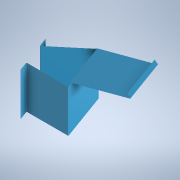
# Autodesk Inventor part: Silla2
Saved by Autodesk Inventor 2022 (Build 260153000, 153)
## iProperties
Created: 2023-10-21
Part Number: Silla2
Material: Generic
Document SubType Name: Sheet Metal
Designer: Administrador
Density: 1 g/cm^3
Sheet Metal Rule: Default
Appearance: Sky Blue Dark
Flat Pattern Width: 113.2 cm
Flat Pattern Length: 180 cm
Flat Pattern Area: 20376 cm^2
Sheet Metal Width: 1132.000 mm
Sheet Metal Length: 1800.000 mm
Sheet Metal Area: 2037600.000 mm^2
Author: Administrador
Autodesk Inventor part; units mm, degrees
ref_plane "YZ Plane" through (0, 0, 0) normal (1, 0, 0) x (0, 1, 0)
ref_plane "XZ Plane" through (0, 0, 0) normal (0, 1, 0) x (-1, 0, 0)
ref_plane "XY Plane" through (0, 0, 0) normal (0, 0, 1) x (1, 0, 0)
sketch "Sketch1" plane through (0, 0, 0) normal (0, 0, 1) x (1, 0, 0)
  point P0 (0, 0)
sketch "Sketch2" plane through (0, 0, 0) normal (0, 0, 1) x (1, 0, 0)
  line L0 (0, 0) -> (1800, 0)
  line L1 (1800, 0) -> (1800, 500)
  line L2 (1800, 500) -> (0, 500)
  line L3 (0, 500) -> (0, 0)
  line L4 (900, 500) -> (900, 0)
  line L5 (900, 500) -> (1170, 500)
  line L6 (1170, 500) -> (630, 500)
  line L7 (630, 500) -> (630, 1132)
  line L8 (630, 1132) -> (1170, 1132)
  line L9 (1170, 1132) -> (1170, 500)
  line L10 (630, 500) -> (630, 520)
  line L11 (630, 520) -> (610, 520)
  arc A0 (610, 500) -> (630, 520) centre (610, 520) ccw
  arc A1 (1170, 520) -> (1190, 500) centre (1190, 520) ccw
  line L12 (610, 500) -> (630, 500)
  line L13 (630, 520) -> (630, 500)
  line L14 (1170, 520) -> (1170, 500)
  line L15 (1190, 500) -> (1170, 500)
  dimension "d0" = 1800
  dimension "d1" = 500
  dimension "d32" = 270
  dimension "d33" = 540
  dimension "d34" = 632
  dimension "d49" = 20
  dimension "d50" = 20
  measures "d0" distance of L0.start L0.end
  measures "d1" distance of L0.end L1.end
  measures "d32" distance of L4.start L5.end
  measures "d33" distance of L7.end L8.end
  measures "d34" distance of L6.end L7.end
  measures "d49" distance of L6.end L10.end
  measures "d50" distance of L10.end L11.end
extrude "Plate1" add sketch "Sketch2" along normal blind 3.048
sketch "Sketch3" plane through (0, 0, 3.048) normal (0, 0, 1) x (1, 0, 0)
  line L0 (1800, 500) -> (0, 500) projected
  line L1 (900, 500) -> (900, 0)
  line L2 (0, 0) -> (1800, 0) projected
  line L3 (900, 0) -> (600, 0)
  line L4 (600, 0) -> (600, 500)
  line L5 (600, 0) -> (110, 0)
  line L6 (0, 500) -> (0, 0) projected
  line L7 (110, 0) -> (0, 0)
  line L8 (110, 0) -> (110, 500)
  line L9 (1200, 0) -> (1200, 500)
  line L10 (1690, 0) -> (1690, 500)
  dimension "d3" = 300
  dimension "d4" = 490
  constraints: 16 end point, 4 symmetric about line, 3 perpendicular, 2 midpoint, 2 point on line, 1 collinear
  measures "d3" distance of L1.end L3.end
  measures "d4" distance of L3.end L5.end
fold "Fold1" angle 110 bend radius 3.048 thickness 3.048 k factor 0.44 line from (110, 0, 3.048) to (110, 500, 3.048) line at bend centre moving side (-1, 0, 0) folds toward (0, 0, 1)
fold "Fold2" angle 110 bend radius 3.048 thickness 3.048 k factor 0.44 line from (600, 0, 3.048) to (600, 500, 3.048) line at bend centre moving side (1, 0, 0) folds toward (0, 0, -1)
sketch "Sketch4" plane through (192.532, 0, -1128.8049) normal (0.9396926, 0, -0.3420201) x (-0.3420201, 0, -0.9396926)
  line L0 (0, 0) -> (0, 500) projected
  line L1 (0, 0) -> (-110, 0)
  line L2 (-1195.7867, 0) -> (0, 0) projected
  line L3 (-110, 0) -> (-600, 0)
  line L4 (-600, 0) -> (-600, 500)
  line L5 (0, 500) -> (-1195.7867, 500) projected
  line L6 (-110, 0) -> (-110, 500)
  point P0 (-994.8799, 0)
  dimension "d17" = 110
  dimension "d18" = 490
  dimension "d19" = 90
  constraints: 8 end point, 4 point on line, 1 vertical
  measures "d17" distance of L0.start L1.end
  measures "d18" distance of L1.end L3.end
  measures "d19" angle of L3 L4
fold "Fold3" angle 110 bend radius 3.048 thickness 3.048 k factor 0.44 line from (230.1542, 0, -1025.4387) to (230.1542, 500, -1025.4387) line at bend centre moving side (-0.3420201, 0, -0.9396926) folds toward (0.9396926, 0, -0.3420201)
fold "Fold4" angle 110 bend radius 3.048 thickness 3.048 k factor 0.44 line from (397.744, 0, -564.9894) to (397.744, 500, -564.9894) line at bend centre moving side (-0.3420201, 0, -0.9396926) folds toward (-0.9396926, 0, 0.3420201)
sketch "Sketch5" plane through (147.5303, 0, 106.5455) normal (0.9396926, 0, -0.3420201) x (-0.3420201, 0, -0.9396926)
  point P0 (150.5783, 0)
ref_plane "Work Plane1" through (-28.7668, 524.6008, -377.8268) normal (0.9396926, 0, -0.3420201) x (0, 1, 0)
sketch "Sketch8" plane through (408.0046, 520, -536.7986) normal (0.9396926, 0, -0.3420201) x (-0.3420201, 0, -0.9396926)
  line L0 (-540, 0) -> (-540, 5)
  line L1 (-540, 612) -> (-540, 0) projected
  line L2 (-540, 5) -> (0, 5)
  line L3 (0, 0) -> (0, 612) projected
  point P0 (-364.8799, -520)
  dimension "d51" = 5
  constraints: 4 end point, 2 point on line, 1 perpendicular
  measures "d51" distance of L0.start L0.end
fold "Fold7" angle 90 bend radius 3.048 thickness 3.048 k factor 0.44 line from (592.6955, 525, -29.3646) to (408.0046, 525, -536.7986) line at bend centre moving side (0, 1, 0) folds toward (0.9396926, 0, -0.3420201)
sketch "Sketch9" plane through (410.8688, 524.6008, -537.8411) normal (0, -1, 0) x (0.9396926, 0, -0.3420201)
  line L0 (603.5528, 540) -> (0, 540) projected
  line L1 (603.5528, 540) -> (553.5528, 540)
  line L2 (553.5528, 540) -> (553.5528, 0)
  line L3 (603.5528, 0) -> (0, 0) projected
  point P0 (-570.0429, 364.8799)
  dimension "d58" = 50
  constraints: 4 end point, 2 point on line, 1 perpendicular
  measures "d58" distance of L0.start L1.end
fold "Fold8" angle 130 bend radius 3.048 thickness 3.048 k factor 0.44 line from (1115.7292, 524.6008, -219.7333) to (931.0383, 524.6008, -727.1673) line at bend centre moving side (0.9396926, 0, -0.3420201) folds toward (0, 1, 0)
equation "\"d2\" = Thickness"
equation "\"d5\" = BendReliefWidth"
equation "\"d6\" = BendReliefDepth"
equation "\"d7\" = MinimumRemnant"
equation "\"d8\" = TransitionRadius"
equation "\"d10\" = BendRadius"
equation "\"d11\" = BendReliefWidth"
equation "\"d12\" = BendReliefDepth"
equation "\"d13\" = MinimumRemnant"
equation "\"d14\" = TransitionRadius"
equation "\"d16\" = BendRadius"
equation "\"d20\" = BendReliefWidth"
equation "\"d21\" = BendReliefDepth"
equation "\"d22\" = MinimumRemnant"
equation "\"d23\" = TransitionRadius"
equation "\"d25\" = BendRadius"
equation "\"d26\" = BendReliefWidth"
equation "\"d27\" = BendReliefDepth"
equation "\"d28\" = MinimumRemnant"
equation "\"d29\" = TransitionRadius"
equation "\"d31\" = BendRadius"
equation "\"d52\" = BendReliefWidth"
equation "\"d53\" = BendReliefDepth"
equation "\"d54\" = MinimumRemnant"
equation "\"d55\" = TransitionRadius"
equation "\"d57\" = BendRadius"
equation "\"d59\" = BendReliefWidth"
equation "\"d60\" = BendReliefDepth"
equation "\"d61\" = MinimumRemnant"
equation "\"d62\" = TransitionRadius"
equation "\"d64\" = BendRadius"
equation "\"BendRadius\" = Thickness"
equation "\"BendReliefWidth\" = Thickness"
equation "\"BendReliefDepth\" = 0.5 * Thickness"
equation "\"CornerReliefSize\" = 4 * Thickness"
equation "\"MinimumRemnant\" = 2 * Thickness"
equation "\"TransitionRadius\" = BendRadius"
equation "\"JacobiRadiusSize\" = BendRadius"
equation "\"GapSize\" = Thickness"
equation "\"Thickness\" = 3.048"
body "Solid1"
